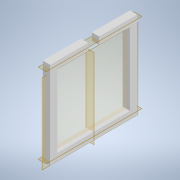
# Autodesk Inventor part: Head Post Holder_Prototype
Saved by Autodesk Inventor 2022 (Build 260153000, 153)
## iProperties
Created: 2022-01-21
Part Number: Head Post Holder_Prototype
Material: Generic
Document SubType Name: Modeling
Designer: gnzak
Density: 1 g/cm^3
Appearance: Default
Author: gnzak
Comments: Cross-sectional Area: 9.625 in^2 Volume: 4.813 in^3 Density of Alumnimum: 0.097 lb/in^3 Approximate Weight: 0.469 lb
Autodesk Inventor part; units mm, degrees
ref_plane "YZ Plane" through (0, 0, 0) normal (1, 0, 0) x (0, 1, 0)
ref_plane "XZ Plane" through (0, 0, 0) normal (0, 1, 0) x (-1, 0, 0)
ref_plane "XY Plane" through (0, 0, 0) normal (0, 0, 1) x (1, 0, 0)
sketch "Sketch1" plane through (0, 0, 0) normal (1, 0, 0) x (0, 1, 0)
  line L0 (83.9305, 131.4309) -> (83.9305, 64.7559)
  line L1 (83.9305, 64.7559) -> (71.2305, 64.7559)
  line L2 (71.2305, 64.7559) -> (71.2305, 118.7309)
  line L3 (71.2305, 118.7309) -> (-55.7695, 118.7309)
  line L4 (-55.7695, 118.7309) -> (-55.7695, -8.2691)
  line L5 (-55.7695, -8.2691) -> (71.2305, -8.2691)
  line L6 (71.2305, -8.2691) -> (71.2305, 45.7059)
  line L7 (71.2305, 45.7059) -> (83.9305, 45.7059)
  line L8 (83.9305, 45.7059) -> (83.9305, -20.9691)
  line L9 (83.9305, -20.9691) -> (-68.4695, -20.9691)
  line L10 (83.9305, 131.4309) -> (-68.4695, 131.4309)
  line L11 (-68.4695, 131.4309) -> (-68.4695, -20.9691)
  dimension "d7" = 152.4
  dimension "d8" = 19.05
  dimension "d9" = 66.675
  dimension "d10" = 152.4
  dimension "d11" = 12.7
  dimension "d12" = 12.7
  dimension "d13" = 12.7
  dimension "d14" = 12.7
  constraints: 24 end point, 8 perpendicular, 4 point on line, 1 horizontal, 1 vertical
  measures "d7" distance of L10.end L9.end
  measures "d8" distance between parallel lines of L7 L1
  measures "d9" distance of L0.start L0.end
  measures "d10" distance of L0.start L10.end
  measures "d11" distance between parallel lines of L4 L11
  measures "d12" distance between parallel lines of L10 L3
  measures "d13" distance between parallel lines of L9 L5
  measures "d14" distance between parallel lines of L8 L6
extrude "Extrusion1" add sketch "Sketch1" along normal blind 12.7
ref_plane "Work Plane1" through (0, -68.4695, 55.2309) normal (0, 0, 1) x (1, 0, 0)
ref_plane "Work Plane2" through (0, 77.5805, 131.4309) normal (0, 1, 0) x (1, 0, 0)
ref_plane "Work Plane3" through (0, -62.1195, 118.7309) normal (0, 1, 0) x (1, 0, 0)
ref_plane "Work Plane4" through (6.35, 0, 0) normal (1, 0, 0) x (0, 0, -1)
equation "\"d9\" = -0.5 * d8 + 0.5 * d7"
equation "\"d12\" = d11"
equation "\"d13\" = d11"
equation "\"d14\" = d11"
body "Solid1"
